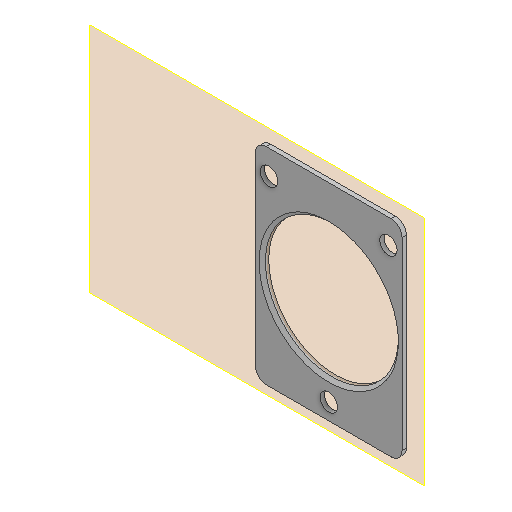
# Autodesk Inventor part: 30_Cube_Insert_Filter_Revolver_Filter_lid
Saved by Autodesk Inventor 2022 (Build 260153000, 153)
## iProperties
Created: 2021-12-19
Part Number: 30_Cube_Insert_Filter_Revolver_Filter_lid
Material: Generisch
Document SubType Name: Modeling
Designer: diederichbenedict
Density: 1 g/cm^3
Appearance: Vorgabe
Author: diederichbenedict
Autodesk Inventor part; units mm, degrees
ref_plane "YZ Plane" through (0, 0, 0) normal (1, 0, 0) x (0, 1, 0)
ref_plane "XZ Plane" through (0, 0, 0) normal (0, 1, 0) x (-1, 0, 0)
ref_plane "XY Plane" through (0, 0, 0) normal (0, 0, 1) x (1, 0, 0)
ref_plane "Arbeitsebene1" through (0, 0, 0) normal (0, 0, 1) x (1, 0, 0)
sketch "Skizze1" plane through (0, 0, 0) normal (0, 0, 1) x (1, 0, 0)
  circle A0 centre (-25, 33.9454) radius 1.4 projected
  circle A1 centre (-3, 33.9454) radius 1.4 projected
  circle A2 centre (-14, 3.4454) radius 1.4 projected
  arc A3 (-19.5678, 31.1928) -> (-19.5678, 7.6981) centre (-14, 19.4454) ccw construction
  line L0 (-2.5, 0.4454) -> (-25.5, 0.4454)
  line L1 (-27.5, 2.4454) -> (-27.5, 36.4454)
  line L2 (-25.5, 38.4454) -> (-2.5, 38.4454)
  line L3 (-0.5, 36.4454) -> (-0.5, 2.4454)
  line L4 (-0.5, 0.4454) -> (-27.5, 38.4454) construction
  line L5 (-27.5, 0.4454) -> (-0.5, 38.4454) construction
  circle A4 centre (-14, 19.4454) radius 12.25
  circle A5 centre (-25, 33.9454) radius 1.63
  circle A6 centre (-14, 3.4454) radius 1.6
  circle A7 centre (-3, 33.9454) radius 1.6
  arc A8 (-25.5, 38.4454) -> (-27.5, 36.4454) centre (-25.5, 36.4454) ccw
  arc A9 (-0.5, 36.4454) -> (-2.5, 38.4454) centre (-2.5, 36.4454) ccw
  arc A10 (-2.5, 0.4454) -> (-0.5, 2.4454) centre (-2.5, 2.4454) ccw
  arc A11 (-27.5, 2.4454) -> (-25.5, 0.4454) centre (-25.5, 2.4454) ccw
  point P0 (0, 0)
  dimension "d0" = 27
  dimension "d1" = 38
  dimension "d2" = 24.5
  dimension "d3" = 0.23
  dimension "d5" = 0.2
  dimension "d6" = 0.2
  dimension "d7" = 2
  constraints: 12 end point, 8 centre point, 8 point on circle, 8 point on line, 8 tangent, 3 equal radius, 2 midpoint, 2 parallel, 1 coincident, 1 horizontal, 1 perpendicular
  measures "d0" distance of L4.end L5.end
  measures "d1" distance of L5.start L4.end
  measures "d2" diameter of A4
  measures "d3" radial gap between concentric circles of A0 A5
  measures "d5" radial gap between concentric circles of A2 A6
  measures "d6" radial gap between concentric circles of A1 A7
  measures "d7" radius of A8
extrude "Extrusion1" add sketch "Skizze1" along normal blind 0.8 contours L0 A11 L1 A8 L2 A9 L3 A10
chamfer "Fase1" distance 0.58 angle 45 1 edges at (-26.25, 19.4454, 0.8)
sketch "Skizze2" plane through (0, 0, 0) normal (0, 0, -1) x (-1, 0, 0)
  circle A0 centre (14, 19.4454) radius 12.25 projected
  circle A1 centre (14, 19.4454) radius 12.75
  point P0 (0, 0)
  dimension "d13" = 0.5
  constraints: 1 centre point
  measures "d13" radial gap between concentric circles of A0 A1
extrude "Extrusion2" add sketch "Skizze2" along normal blind 0.4
